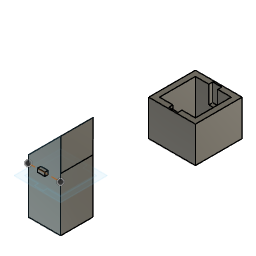
Reader (Autodesk Fusion 360 design; units mm, degrees)
Autodesk Fusion 360 part; units mm, degrees
sketch "Sketch1" plane through (0, 0, 0) normal (0, 1, 0) x (1, 0, 0)
  line L0 (0, 0) -> (25.4, 0)
  line L1 (25.4, 0) -> (25.4, -38.1)
  line L2 (25.4, -38.1) -> (0, -38.1)
  line L3 (0, -38.1) -> (0, 0)
  line L4 (25.4, -38.1) -> (25.4, -63.5)
  line L5 (25.4, -63.5) -> (0, -38.1)
  constraint horizontal L0
  constraint vertical L1
  constraint horizontal L2
  constraint vertical L3
  constraint coincident L0.start L3.end
  constraint perpendicular L2 L4
sketch "Sketch2" plane through (0, 0, 0) normal (0, -1, 0) x (1, 0, 0)
  line L0 (25.4, 0) -> (25.4, 63.5)
  line L1 (25.4, 63.5) -> (0, 38.1)
  line L2 (0, 38.1) -> (0, 0)
  line L3 (0, 0) -> (25.4, 0)
  line L4 (15.875, 39.37) -> (9.525, 39.37)
  line L5 (9.525, 39.37) -> (9.525, 36.83)
  line L6 (9.525, 36.83) -> (15.875, 36.83)
  line L7 (15.875, 36.83) -> (15.875, 39.37)
  line L8 (15.875, 39.37) -> (9.525, 36.83) construction
  line L9 (9.525, 39.37) -> (15.875, 36.83) construction
  point P0 (12.7, 38.1)
  dimension "d3" = 6.35
  constraint horizontal L4
  constraint perpendicular L4 L5
  constraint parallel L4 L6
  constraint parallel L5 L7
  constraint coincident L8 P0
  constraint coincident L9 P0
  measures "d3" distance of L5.end L6.end
sketch "Sketch3" plane through (0, 25.4, 0) normal (0, 1, 0) x (-1, 0, 0)
  line L0 (-25.4, 63.5) -> (-25.4, 0)
  line L1 (-25.4, 0) -> (0, 0)
  line L2 (0, 0) -> (0, 38.1)
  line L3 (0, 38.1) -> (-25.4, 63.5)
  line L4 (-9.525, 39.37) -> (-15.875, 39.37)
  line L5 (-15.875, 39.37) -> (-15.875, 36.83)
  line L6 (-15.875, 36.83) -> (-9.525, 36.83)
  line L7 (-9.525, 36.83) -> (-9.525, 39.37)
  line L8 (-9.525, 39.37) -> (-15.875, 36.83) construction
  line L9 (-15.875, 39.37) -> (-9.525, 36.83) construction
  point P0 (-12.7, 38.1)
  dimension "d6" = 6.35
  dimension "d7" = 2.54
  dimension "d47" = 25.4
  constraint horizontal L4
  constraint perpendicular L4 L5
  constraint parallel L4 L6
  constraint parallel L5 L7
  constraint coincident L8 P0
  constraint coincident L9 P0
  measures "d6" distance of L5.end L6.end
  measures "d7" distance of L4.end L5.end
  measures "d47" distance of L0.end L1.end
sketch "Sketch4" plane through (0, 0, 0) normal (0, 0, 1) x (1, 0, 0)
  line L0 (-2.54, -2.54) -> (27.94, -2.54)
  line L1 (27.94, -2.54) -> (27.94, 27.94)
  line L2 (27.94, 27.94) -> (-2.54, 27.94)
  line L3 (-2.54, 27.94) -> (-2.54, -2.54)
  constraint horizontal L0
  constraint vertical L1
  constraint horizontal L2
  constraint vertical L3
sketch "Sketch6" plane through (0, 0, 0) normal (0, 0, 1) x (1, 0, 0)
  line L0 (-3.81, 29.21) -> (29.21, 29.21)
  line L1 (29.21, 29.21) -> (29.21, -3.81)
  line L2 (29.21, -3.81) -> (-3.81, -3.81)
  line L3 (-3.81, -3.81) -> (-3.81, 29.21)
  line L4 (15.875, 0) -> (15.875, -2.54)
  line L5 (9.525, 27.94) -> (15.875, 27.94)
  line L6 (15.875, -2.54) -> (9.525, -2.54)
  line L7 (0, 0) -> (0, 25.4)
  line L8 (25.4, 0) -> (25.4, 25.4)
  dimension "d14" = 33.02
  dimension "d15" = 33.02
  dimension "d16" = 2.54
  dimension "d17" = 1.27
  dimension "d18" = 1.27
  dimension "d19" = 3.81
  dimension "d20" = 3.81
  constraint horizontal L0
  constraint vertical L1
  constraint horizontal L2
  constraint vertical L3
  measures "d14" distance of L0.start L0.end
  measures "d15" distance of L0.start L2.end
  measures "d16" distance of L4.start L4.end
  measures "d17" distance of L0 L5
  measures "d18" distance of L2 L6
  measures "d19" distance of L3 L7
  measures "d20" distance of L1 L8
move_body "Move2" [no effect]
sketch "Sketch11" plane through (0, 0, 0) normal (0, 0, 1) x (1, 0, 0)
  line L0 (0, 0) -> (33.02, 0)
  line L1 (33.02, 0) -> (33.02, 33.02)
  line L2 (33.02, 33.02) -> (0, 33.02)
  line L3 (0, 33.02) -> (0, 0)
  dimension "d35" = 33.02
  dimension "d36" = 33.02
  constraint horizontal L0
  constraint vertical L1
  constraint horizontal L2
  constraint vertical L3
  constraint coincident L0.start L3.end
  measures "d35" distance of L1.end L2.end
  measures "d36" distance of L0.start L2.end
extrude "Extrude10" add sketch "Sketch11" along normal blind 25.4 makes body 1
sketch "Sketch12" plane through (0, 0, 25.4) normal (0, 0, 1) x (-1, 0, 0)
  line L0 (0, -33.02) -> (0, 0)
  line L1 (0, 0) -> (-33.02, 0)
  line L2 (-33.02, 0) -> (-33.02, -33.02)
  line L3 (-33.02, -33.02) -> (0, -33.02)
  line L4 (-29.21, -29.21) -> (-3.81, -29.21)
  line L5 (-3.81, -29.21) -> (-3.81, -3.81)
  line L6 (-3.81, -3.81) -> (-29.21, -3.81)
  line L7 (-29.21, -3.81) -> (-29.21, -29.21)
  line L8 (-29.21, -29.21) -> (-3.81, -3.81) construction
  line L9 (-3.81, -29.21) -> (-29.21, -3.81) construction
  point P0 (-16.51, -16.51)
  dimension "d39" = 25.4
  dimension "d40" = 25.4
  constraint horizontal L4
  constraint perpendicular L4 L5
  constraint parallel L4 L6
  constraint parallel L5 L7
  constraint coincident L8 P0
  constraint coincident L9 P0
  measures "d39" distance of L5.end L6.end
  measures "d40" distance of L4.end L5.end
extrude "Extrude11" cut sketch "Sketch12" against normal blind 45.72 contours L4 L5 L6 L7 bodies 1
sketch "Sketch13" plane through (0, 0, 25.4) normal (0, 0, 1) x (-1, 0, 0)
  line L0 (-3.81, -29.21) -> (-29.21, -29.21)
  line L1 (-29.21, -29.21) -> (-29.21, -3.81)
  line L2 (-29.21, -3.81) -> (-3.81, -3.81)
  line L3 (-3.81, -3.81) -> (-3.81, -29.21)
  line L4 (0, -33.02) -> (0, 0)
  line L5 (0, 0) -> (-33.02, 0)
  line L6 (-33.02, 0) -> (-33.02, -33.02)
  line L7 (-33.02, -33.02) -> (0, -33.02)
  line L8 (-16.51, -3.81) -> (-13.335, -3.81)
  line L9 (-13.335, -3.81) -> (-13.335, -1.016)
  line L10 (-13.335, -1.016) -> (-16.51, -1.016)
  line L11 (-16.51, -1.016) -> (-16.51, -3.81)
  line L12 (-19.685, -1.016) -> (-16.51, -1.016)
  line L13 (-19.685, -3.81) -> (-19.685, -1.016)
  line L14 (-16.51, -3.81) -> (-19.685, -3.81)
  line L15 (-16.51, -29.21) -> (-13.335, -29.21)
  line L16 (-16.51, -29.21) -> (-19.685, -29.21)
  line L17 (-19.685, -32.004) -> (-16.51, -32.004)
  line L18 (-13.335, -32.004) -> (-16.51, -32.004)
  line L19 (-13.335, -29.21) -> (-13.335, -32.004)
  line L20 (-16.51, -32.004) -> (-16.51, -29.21)
  line L21 (-19.685, -29.21) -> (-19.685, -32.004)
  dimension "d43" = 3.175
  dimension "d44" = 2.794
  constraint horizontal L8
  constraint vertical L9
  constraint horizontal L10
  constraint vertical L11
  constraint midpoint L2 L8.start
  constraint symmetric L8.start L11 L14.start
  constraint symmetric L8.end L11 L13.start
  constraint symmetric L9.end L11 L12.start
  constraint symmetric L10.end L11 L12.end
  measures "d43" distance of L8.start L8.end
  measures "d44" distance of L8.start L10.end
extrude "Extrude12" cut sketch "Sketch13" against normal blind 12.7 contours L0 L15 L18 L19 L20 | L0 L16 L17 L20 L21 | L2 L8 L9 L10 L11 | L2 L11 L12 L13 L14 bodies 1
sketch "Sketch14" plane through (0, 0, 0) normal (0, 1, 0) x (1, 0, 0)
  line L0 (27.94, 0) -> (5.08, 0)
  line L1 (5.08, 0) -> (5.08, -38.1)
  line L2 (5.08, -38.1) -> (27.94, -38.1)
  line L3 (27.94, -38.1) -> (27.94, 0)
  line L4 (5.08, -38.1) -> (28.0867, -61.1067)
  line L5 (5.08, -38.1) -> (37.6164, -38.1) construction
  line L6 (28.0867, -61.1067) -> (27.94, -38.1)
  dimension "d48" = 22.86
  dimension "d49" = 38.1
  dimension "d50" = 45
  constraint horizontal L0
  constraint vertical L1
  constraint horizontal L2
  constraint vertical L3
  constraint horizontal L5
  measures "d48" distance of L0.start L0.end
  measures "d49" distance of L0.start L2.end
  measures "d50" angle of L4 L5
extrude "Extrude13" add sketch "Sketch14" along normal blind 22.86 separate body makes body 2
move_body "Move3" bodies 2 to x (1, 0, 0) y (0, 1, 0) z (0, 0, 1) at (0, 60.96, 0)
sketch "Sketch15" plane through (0, 60.96, 0) normal (0, -1, 0) x (1, 0, 0)
  line L0 (27.94, 38.1) -> (28.0867, 61.1067)
  line L1 (28.0867, 61.1067) -> (5.08, 38.1)
  line L2 (5.08, 38.1) -> (5.08, 0)
  line L3 (5.08, 0) -> (27.94, 0)
  line L4 (27.94, 0) -> (27.94, 38.1)
  line L5 (5.08, 38.1) -> (27.94, 38.1)
  line L6 (19.05, 35.56) -> (13.97, 35.56)
  line L7 (13.97, 35.56) -> (13.97, 33.02)
  line L8 (13.97, 33.02) -> (19.05, 33.02)
  line L9 (19.05, 33.02) -> (19.05, 35.56)
  line L10 (19.05, 35.56) -> (13.97, 33.02) construction
  line L11 (13.97, 35.56) -> (19.05, 33.02) construction
  line L12 (5.08, 38.1) -> (37.6164, 38.1)
  point P0 (16.51, 34.29)
  dimension "d54" = 5.08
  dimension "d55" = 2.54
  dimension "d60" = 2.54
  constraint coincident L1.end L2.start
  constraint coincident L0.start L4.end
  constraint horizontal L6
  constraint perpendicular L6 L7
  constraint parallel L6 L8
  constraint parallel L7 L9
  constraint coincident L10 P0
  constraint coincident L11 P0
  measures "d54" distance of L7.end L8.end
  measures "d55" distance of L6.end L7.end
  measures "d60" distance of L6 L12
extrude "Extrude14" add sketch "Sketch15" along normal blind 2.286 contours L6 L7 L8 L9 bodies 2
sketch "Sketch16" plane through (0, 83.82, 0) normal (0, 1, 0) x (-1, 0, 0)
  line L0 (-28.0867, 61.1067) -> (-27.94, 38.1)
  line L1 (-27.94, 38.1) -> (-27.94, 0)
  line L2 (-27.94, 0) -> (-5.08, 0)
  line L3 (-5.08, 0) -> (-5.08, 38.1)
  line L4 (-5.08, 38.1) -> (-28.0867, 61.1067)
  line L5 (-5.08, 38.1) -> (-27.94, 38.1)
  line L6 (-13.97, 35.56) -> (-19.05, 35.56)
  line L7 (-19.05, 35.56) -> (-19.05, 33.02)
  line L8 (-19.05, 33.02) -> (-13.97, 33.02)
  line L9 (-13.97, 33.02) -> (-13.97, 35.56)
  line L10 (-13.97, 35.56) -> (-19.05, 33.02) construction
  line L11 (-19.05, 35.56) -> (-13.97, 33.02) construction
  point P0 (-16.51, 34.29)
  dimension "d58" = 5.08
  dimension "d59" = 2.54
  dimension "d61" = 2.54
  constraint coincident L3.end L4.start
  constraint coincident L0.end L1.start
  constraint horizontal L6
  constraint perpendicular L6 L7
  constraint parallel L6 L8
  constraint parallel L7 L9
  constraint coincident L10 P0
  constraint coincident L11 P0
  measures "d58" distance of L7.end L8.end
  measures "d59" distance of L6.end L7.end
  measures "d61" distance of L5 L6
extrude "Extrude15" add sketch "Sketch16" along normal blind 2.286 contours L6 L7 L8 L9 bodies 2
copy_body "Body->Comp1" bodies 2 removing the originals makes body 3 in component "ReaderBodyComponent"
copy_body "Body->Comp2" bodies 1 removing the originals makes body 4 in component "ReaderContainerComponent"
move_body "Move1" bodies 3 to x (1, 0, 0) y (0, 1, 0) z (0, 0, 1) at (0, -55.88, 0) in component "ReaderBodyComponent"
sketch "Sketch17" plane through (-16.51, 0, 16.51) normal (-0.707107, 0, 0.707107) x (0, -1, 0)
  line L0 (-5.08, 30.5329) -> (-5.08, 63.0693)
  line L1 (-5.08, 63.0693) -> (-27.94, 63.0693)
  line L2 (-27.94, 63.0693) -> (-27.94, 30.5329)
  line L3 (-27.94, 30.5329) -> (-5.08, 30.5329)
sketch "Sketch18" plane through (0, 0, 25.4) normal (0, 0, 1) x (-1, 0, 0)
  line L0 (-19.685, -32.004) -> (-19.685, -29.21)
  line L1 (-19.685, -29.21) -> (-29.21, -29.21)
  line L2 (-29.21, -29.21) -> (-29.21, -3.81)
  line L3 (-29.21, -3.81) -> (-19.685, -3.81)
  line L4 (-19.685, -3.81) -> (-19.685, -1.016)
  line L5 (-19.685, -1.016) -> (-13.335, -1.016)
  line L6 (-13.335, -1.016) -> (-13.335, -3.81)
  line L7 (-13.335, -3.81) -> (-3.81, -3.81)
  line L8 (-3.81, -3.81) -> (-3.81, -29.21)
  line L9 (-3.81, -29.21) -> (-13.335, -29.21)
  line L10 (-13.335, -29.21) -> (-13.335, -32.004)
  line L11 (-13.335, -32.004) -> (-19.685, -32.004)
  line L12 (0, -33.02) -> (0, 0)
  line L13 (0, 0) -> (-33.02, 0)
  line L14 (-33.02, 0) -> (-33.02, -33.02)
  line L15 (-33.02, -33.02) -> (0, -33.02)
sketch "Sketch19" plane through (0, 5.08, 0) normal (0, -1, 0) x (1, 0, 0)
  line L0 (19.05, 33.02) -> (13.97, 33.02)
  line L1 (13.97, 33.02) -> (13.97, 35.56)
  line L2 (13.97, 35.56) -> (19.05, 35.56)
  line L3 (19.05, 35.56) -> (19.05, 33.02)
  line L4 (27.94, 38.1) -> (28.0867, 61.1067)
  line L5 (28.0867, 61.1067) -> (5.08, 38.1)
  line L6 (5.08, 38.1) -> (5.08, 0)
  line L7 (5.08, 0) -> (27.94, 0)
  line L8 (27.94, 0) -> (27.94, 38.1)
  line L9 (27.94, 33.02) -> (5.08, 33.02) construction
  constraint coincident L8 L9.start
  constraint coincident L6 L9.end
  constraint perpendicular L6 L9
component "ReaderBodyComponent" placed x (1, 0, 0) y (0, 1, 0) z (0, 0, 1) at (0, 0, 0)
component "ReaderContainerComponent" placed x (1, 0, 0) y (0, 1, 0) z (0, 0, 1) at (-0.3806, 95.7718, 0)
named bodies: "ReaderContainer"
